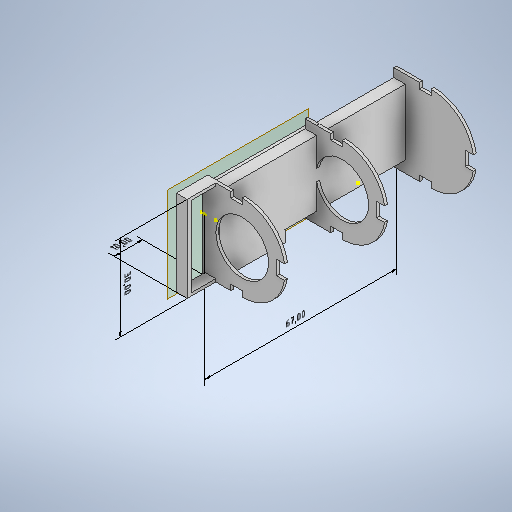
# Autodesk Inventor part: Part4
Saved by Autodesk Inventor 2025.3 (Build 293356000, 356)
## iProperties
Created: 2025-06-07
Part Number: Part4
Material: Generic
Document SubType Name: Modeling
Designer: Repete
Density: 1 g/cm^3
Appearance: Default
Author: Repete
Autodesk Inventor part; units mm, degrees
ref_plane "YZ Plane" through (0, 0, 0) normal (1, 0, 0) x (0, 1, 0)
ref_plane "XZ Plane" through (0, 0, 0) normal (0, 1, 0) x (-1, 0, 0)
ref_plane "XY Plane" through (0, 0, 0) normal (0, 0, 1) x (1, 0, 0)
sketch "Sketch1" plane through (0, 0, 0) normal (0, 1, 0) x (-1, 0, 0)
  circle A0 centre (4.6316, -3.7972) radius 9.2
  line L0 (17.6316, 11.2028) -> (4.6316, 11.2028)
  line L1 (4.6316, -18.7972) -> (17.6316, -18.7972)
  line L2 (17.6316, -18.7972) -> (17.6316, 11.2028)
  arc A1 (4.6316, 11.2028) -> (-10.1586, -1.2972) centre (4.6316, -3.7972) ccw
  arc A2 (-10.1586, -6.2972) -> (4.6316, -18.7972) centre (4.6316, -3.7972) ccw
  arc A3 (-10.1586, -1.2972) -> (-10.1586, -6.2972) centre (4.6316, -3.7972) ccw
  point P0 (17.6316, -3.7972)
  dimension "d6" = 30
  dimension "d7" = 18.4
  dimension "d13" = 13
  constraints: 6 end point, 6 point on circle, 4 centre point, 2 concentric, 1 coincident, 1 horizontal, 1 midpoint, 1 parallel
  measures "d6" distance of L1.end L0.start
  measures "d7" diameter of A0
  measures "d13" distance of point (17.632, -3.797) A0.centre
extrude "Extrusion1" add sketch "Sketch1" along normal blind 1
sketch "Sketch5" plane through (0, 1, 0) normal (0, 1, 0) x (1, 0, 0)
  line L0 (-17.6316, 18.7972) -> (-17.6316, -11.2028) projected
  line L1 (-4.6316, 18.7972) -> (-17.6316, 18.7972) projected
  line L2 (-17.6316, -11.2028) -> (-13.6316, -11.2028)
  line L3 (-13.6316, -11.2028) -> (-13.6316, 18.7972)
  line L4 (-13.6316, 18.7972) -> (-17.6316, 18.7972)
  line L5 (-17.6316, 18.7972) -> (-17.6316, -11.2028)
  point P0 (0, 0)
  dimension "d17" = 4
  constraints: 8 end point, 2 parallel, 1 horizontal, 1 perpendicular, 1 point on line
  measures "d17" distance between parallel lines of L0 L3
extrude "Extrusion2" add sketch "Sketch5" along normal blind 35
sketch "Sketch6" plane through (-17.6316, 0, -18.7972) normal (-1, 0, 0) x (0, 0, 1)
  line L0 (0, 0) -> (0, 36) projected
  line L1 (0, 1) -> (25, 1)
  line L2 (25, 1) -> (25, 35)
  line L3 (25, 35) -> (0, 35)
  line L4 (0, 35) -> (0, 1)
  line L5 (0, 0) -> (30, 0) projected
  point P0 (18.7972, 0)
  point P1 (0, 35)
  point P2 (0, 35)
  dimension "d20" = 25
  dimension "d21" = 1
  dimension "d22" = 34
  constraints: 8 end point, 2 parallel, 1 horizontal, 1 perpendicular, 1 point on line
  measures "d20" distance of L1.start L1.end
  measures "d21" distance between parallel lines of L5 L1
  measures "d22" distance between parallel lines of L1 L3
extrude "Extrusion3" cut sketch "Sketch6" against normal blind 3
sketch "Sketch7" plane through (-17.6316, 0, -18.7972) normal (-1, 0, 0) x (0, 0, 1)
  point P0 (18.7972, 0)
sketch "Sketch8" plane through (-17.6316, 0, -18.7972) normal (-1, 0, 0) x (0, 0, 1)
  line L0 (30, 1) -> (30, 36) projected
  line L1 (25, 35) -> (25, 1) projected
  line L2 (30, 15) -> (25, 15)
  line L3 (25, 15) -> (25, 23)
  line L4 (25, 23) -> (30, 23)
  line L5 (30, 23) -> (30, 15)
  line L6 (0, 0) -> (30, 0) projected
  point P0 (18.7972, 0)
  point P1 (27.5, 15)
  point P2 (27.5, 23)
  point P3 (24, 34.5)
  dimension "d27" = 15
  dimension "d28" = 8
  constraints: 8 end point, 2 midpoint, 2 parallel, 1 horizontal, 1 perpendicular, 1 point on line, 2 other
  measures "d27" distance from line of L6 point (27.5, 15)
  measures "d28" distance of point (27.5, 15) point (27.5, 23)
extrude "Extrusion4" [suppressed]
sketch "Sketch9" plane through (-14.6316, 35, 6.2028) normal (0, 0, -1) x (-1, 0, 0)
  line L0 (3, -12) -> (3.5, -12) projected
  line L1 (3, 0) -> (3, -34) projected
  line L2 (3.5, -12) -> (3, -12)
  line L3 (3, -12) -> (3, -20)
  line L4 (3, -20) -> (3.5, -20)
  line L5 (3.5, -20) -> (3.5, -12)
  point P0 (-14.6316, -35)
  constraints: 8 end point, 2 parallel, 1 horizontal, 1 perpendicular
extrude "Extrusion5" [suppressed]
sketch "Sketch12" plane through (-18.1316, 23, 11.2028) normal (0, 1, 0) x (1, 0, 0)
  line L0 (0, 0) -> (0, 22) projected
  line L1 (0.5, 5) -> (0.5, 22) projected
  line L2 (0, 22) -> (0.5, 22)
  line L3 (0.5, 15.462) -> (0, 15.462)
  line L4 (0, 15.462) -> (0, 22)
  line L5 (0.5, 15.462) -> (1.9334, 18.7689)
  line L6 (1.9334, 18.7689) -> (1.9334, 22)
  line L7 (1.9334, 22) -> (0.5, 22)
  point P0 (18.1316, 11.2028)
  dimension "d36" = 0.5
  constraints: 12 end point, 1 horizontal, 1 parallel, 1 perpendicular, 1 point on line, 1 vertical
  measures "d36" distance of L0.end L2.end
extrude "Extrusion6" [suppressed]
fillet "Fillet1" [suppressed]
sketch "Sketch20" plane through (0, 36, 0) normal (0, 1, 0) x (1, 0, 0)
  point P0 (0, 0)
ref_plane "Work Plane1" through (0, 36, 0) normal (0, -1, 0) x (1, 0, 0)
sketch "Sketch24" plane through (-4.6316, 0, -18.7972) normal (0, 0, -1) x (-1, 0, 0)
  line L0 (0, 0) -> (-14.7902, 0) projected
  line L1 (0, 1) -> (9, 1) projected
  line L2 (0, 0) -> (4, 0)
  line L3 (4, 0) -> (4, 1)
  line L4 (4, 1) -> (0, 1)
  line L5 (0, 1) -> (0, 0)
  point P0 (-4.6316, 0)
  dimension "d69" = 4
  constraints: 8 end point, 2 parallel, 1 horizontal, 1 perpendicular, 1 point on line
  measures "d69" distance between parallel lines of L3 L5
extrude "Extrusion16" cut sketch "Sketch24" against normal blind 2
sketch "Sketch25" plane through (-17.6316, 0, 11.2028) normal (0, 0, 1) x (1, 0, 0)
  line L0 (4, 1) -> (13, 1) projected
  line L1 (3.8, 0) -> (22.2, 0) projected
  line L2 (13, 1) -> (9, 1)
  line L3 (9, 1) -> (9, 0)
  line L4 (9, 0) -> (13, 0)
  line L5 (13, 0) -> (13, 1)
  point P0 (17.6316, 0)
  dimension "d72" = 4
  constraints: 8 end point, 2 parallel, 1 horizontal, 1 perpendicular, 1 point on line
  measures "d72" distance between parallel lines of L3 L5
extrude "Extrusion17" cut sketch "Sketch25" against normal blind 2
sketch "Sketch30" plane through (-13.6316, 1, -1.8894) normal (1, 0, 0) x (0, 0, -1)
  point P0 (-1.8894, -1)
sketch "Sketch31" plane through (-13.6316, 1, -1.8894) normal (1, 0, 0) x (0, 0, -1)
  line L0 (-13.0921, 0) -> (-13.0921, 35) projected
  line L1 (16.9079, 0) -> (-13.0921, 0) projected
  line L2 (-13.0921, 34) -> (-10.0921, 34)
  line L3 (-10.0921, 34) -> (-10.0921, 0)
  line L4 (-10.0921, 0) -> (-13.0921, 0)
  line L5 (-13.0921, 0) -> (-13.0921, 34)
  line L6 (-13.0921, 35) -> (16.9079, 35) projected
  point P0 (-1.8894, -1)
  point P1 (-11.5921, 34)
  dimension "d97" = 3
  dimension "d100" = 1
  constraints: 8 end point, 2 parallel, 2 point on line, 1 horizontal, 1 midpoint, 1 perpendicular
  measures "d97" distance of L2.start L2.end
  measures "d100" distance from line of L6 point (-11.592, 34)
extrude "Extrusion22" cut sketch "Sketch31" against normal through all
sketch "Sketch32" plane through (0, 36, 0) normal (0, -1, 0) x (1, 0, 0)
  circle A0 centre (-4.6552, -3.8036) radius 9.2
  line L0 (-17.6552, -18.8036) -> (-8.6316, -18.8036)
  line L1 (-8.6316, 11.1964) -> (-17.6552, 11.1964)
  line L2 (-17.6552, 11.1964) -> (-17.6552, -18.8036)
  arc A1 (-4.6552, -18.8036) -> (10.135, -6.3036) centre (-4.6552, -3.8036) ccw
  arc A2 (10.135, -6.3036) -> (-4.6552, 11.1964) centre (-4.6552, -3.8036) ccw
  line L3 (-4.6316, 9.2028) -> (-4.6316, 11.2028) projected
  line L4 (-4.6316, 9.2028) -> (-8.6316, 9.2028)
  line L5 (-8.6316, 9.2028) -> (-8.6316, 11.1964)
  line L6 (-4.6316, 11.1964) -> (-4.6316, 9.2028)
  line L7 (-4.6316, -16.7972) -> (-8.6316, -16.7972) projected
  line L8 (-8.6316, -16.7972) -> (-4.6316, -16.7972)
  line L9 (-4.6316, -16.7972) -> (-4.6316, -18.8036)
  line L10 (-8.6316, -18.8036) -> (-8.6316, -16.7972)
  arc A3 (10.135, -6.3036) -> (10.135, -6.3036) centre (-3.0684, -4.0718) ccw
  point P0 (0, 0)
  point P1 (-17.6552, -3.8036)
  point P2 (-4.6316, -16.7972)
  point P3 (10.135, -6.3036)
  dimension "d101" = 30
  dimension "d102" = 18.4
  dimension "d103" = 13
  constraints: 18 end point, 8 point on circle, 4 centre point, 3 parallel, 2 horizontal, 2 perpendicular, 1 coincident, 1 midpoint, 1 tangent
  measures "d101" distance of L1.end L0.start
  measures "d102" diameter of A0
  measures "d103" distance of point (-17.655, -3.804) A0.centre
extrude "Extrusion23" add sketch "Sketch32" along normal blind 1 contours L2 L1 L5 L4 A3 L7 L10 L0 | A3 L4 L3 L9 L7 | A3 A1 L9 | L3 A2 A3
ref_plane "Work Plane3" through (0, 66, 0) normal (0, 1, 0) x (1, 0, 0)
sketch "Sketch34" plane through (0, 66, 0) normal (0, 1, 0) x (1, 0, 0)
  line L0 (-17.6552, -11.1991) -> (-8.6316, -11.1991)
  line L1 (-8.6316, 18.8009) -> (-17.6552, 18.8009)
  line L2 (-17.6552, 18.8009) -> (-17.6552, -11.1991)
  arc A0 (-4.6552, -11.1991) -> (10.135, 1.3009) centre (-4.6552, 3.8009) ccw
  arc A1 (10.135, 6.3009) -> (-4.6552, 18.8009) centre (-4.6552, 3.8009) ccw
  line L3 (-4.6316, 16.8009) -> (-8.6316, 16.8009)
  line L4 (-8.6316, 16.8009) -> (-8.6316, 18.8009)
  line L5 (-4.6316, 18.8009) -> (-4.6316, 16.8009)
  line L6 (-8.6316, -9.1991) -> (-4.6316, -9.1991)
  line L7 (-4.6316, -9.1991) -> (-4.6316, -11.1991)
  line L8 (-8.6316, -11.1991) -> (-8.6316, -9.1991)
  arc A2 (10.135, 1.3009) -> (10.135, 6.3009) centre (-4.6552, 3.8009) ccw
  point P0 (0, 0)
  point P1 (-17.6552, 3.8009)
  dimension "d113" = 30
  dimension "d137" = 2
  dimension "d138" = 2
  constraints: 18 end point, 8 point on circle, 3 centre point, 3 parallel, 2 horizontal, 2 perpendicular, 1 midpoint
  measures "d113" distance of L1.end L0.start
  measures "d137" distance between parallel lines of L6 L0
  measures "d138" distance between parallel lines of L1 L3
extrude "Extrusion25" add sketch "Sketch34" along normal blind 1
sketch "Sketch13" plane through (-14.6316, 0, -18.7972) normal (-1, 0, 0) x (0, 0, 1)
  line L0 (0, 35) -> (25, 35) projected
  line L1 (0, 35) -> (4, 35)
  line L2 (4, 35) -> (4, 24)
  line L3 (4, 24) -> (0, 24)
  line L4 (0, 24) -> (0, 35)
  point P0 (18.7972, 0)
  dimension "d37" = 11
  dimension "d38" = 4
  constraints: 8 end point, 2 parallel, 1 horizontal, 1 perpendicular
  measures "d37" distance of L3.end L0.start
  measures "d38" distance of L2.end L3.end
extrude "Extrusion7" cut sketch "Sketch13" along normal through all both and the other way through all
sketch "Sketch33" plane through (0, 36, 0) normal (0, 1, 0) x (1, 0, 0)
  line L0 (-17.6316, -8.2028) -> (-13.6316, -8.2028)
  line L1 (-13.6316, -8.2028) -> (-13.6316, 14.7972)
  line L2 (-13.6316, 14.7972) -> (-14.6316, 14.7972)
  line L3 (-17.6316, -6.2028) -> (-17.6316, -8.2028)
  line L4 (-17.6316, 18.7972) -> (-17.6316, -11.2028) projected
  line L5 (-17.6316, -6.2028) -> (-14.6316, -6.2028)
  line L6 (-14.6316, -6.2028) -> (-14.6316, 14.7972)
  point P0 (0, 0)
  constraints: 12 end point, 2 horizontal, 2 parallel, 2 perpendicular, 2 other
extrude "Extrusion24" add sketch "Sketch33" along normal up to surface (30 mm away)
sketch "Sketch35" plane through (0, 0, 0) normal (0, -1, 0) x (1, 0, 0)
  line L0 (-17.6316, 11.2028) -> (-8.6316, 11.2028) projected
  line L1 (-17.6316, -18.7972) -> (-14.6316, -18.7972) projected
  line L2 (-13.8651, 11.2028) -> (-17.6316, 11.2028)
  line L3 (-17.6316, 11.2028) -> (-17.6316, -18.7972)
  line L4 (-17.6316, -18.7972) -> (-13.8651, -18.7972)
  line L5 (-13.8651, -18.7972) -> (-13.8651, 11.2028)
  point P0 (0, 0)
  constraints: 8 end point, 2 parallel, 1 horizontal, 1 perpendicular, 1 point on line
extrude "Extrusion26" add sketch "Sketch35" along normal blind 10
sketch "Sketch36" plane through (-13.8651, 0, 11.2028) normal (1, 0, 0) x (0, 0, -1)
  line L0 (0, 0) -> (30, 0) projected
  line L1 (1, 0) -> (29, 0)
  line L2 (29, 0) -> (29, -8.5)
  line L3 (29, -8.5) -> (1, -8.5)
  line L4 (1, -8.5) -> (1, 0)
  line L5 (30, 0) -> (30, -10) projected
  line L6 (0, 0) -> (0, -10) projected
  line L7 (30, -10) -> (0, -10) projected
  point P0 (11.2028, 0)
  point P1 (29, 0)
  dimension "d126" = 1
  dimension "d127" = 1
  dimension "d128" = 1.5
  constraints: 8 end point, 2 parallel, 1 horizontal, 1 perpendicular, 1 point on line
  measures "d126" distance between parallel lines of L5 L2
  measures "d127" distance between parallel lines of L6 L4
  measures "d128" distance between parallel lines of L7 L3
extrude "Extrusion27" cut sketch "Sketch36" against normal through all contours L0 L2 L3 L4
sketch "Sketch37" plane through (0, 67, 0) normal (0, 1, 0) x (1, 0, 0)
  line L0 (12.3499, 1.3009) -> (7.3448, 1.3009)
  line L1 (7.3448, 1.3009) -> (7.3448, 6.3009)
  line L2 (7.3448, 6.3009) -> (12.3499, 6.3009)
  line L3 (12.3499, 6.3009) -> (12.3499, 1.3009)
  arc A0 (-4.6316, -11.1991) -> (-4.6316, 18.8009) centre (-4.6552, 3.8009) ccw projected
  line L4 (-4.6316, 16.8009) -> (-8.6316, 16.8009) projected
  point P0 (0, 0)
  point P1 (12.3499, 3.8009)
  point P2 (9.8474, 1.3009)
  point P3 (9.8474, 6.3009)
  dimension "d140" = 5
  dimension "d143" = 10.5
  dimension "d146" = 12
  constraints: 8 end point, 3 midpoint, 2 parallel, 1 horizontal, 1 perpendicular
  measures "d140" distance between parallel lines of L2 L0
  measures "d143" distance from line of point (9.847, 6.301) L4
  measures "d146" distance from line of A0.centre L1
extrude "Extrusion28" cut sketch "Sketch37" against normal through all
ref_plane "Work Plane4" through (-18.6316, 1, 6.2028) normal (-1, 0, 0) x (0, 0, 1)
sketch "Sketch38" plane through (-18.6316, 1, 6.2028) normal (-1, 0, 0) x (0, 0, 1)
  line L0 (5, -1) -> (-7.5036, -1) projected
  line L1 (-25.0064, 35) -> (1.9936, 35)
  line L2 (1.9936, 35) -> (1.9936, -1)
  line L3 (1.9936, -1) -> (-25.0064, -1)
  line L4 (-25.0064, -1) -> (-25.0064, 35)
  point P0 (-6.2028, -1)
  constraints: 8 end point, 2 parallel, 1 horizontal, 1 perpendicular, 1 point on line
extrude "Extrusion29" add sketch "Sketch38" against normal up to surface (1 mm away)
sketch "Sketch39" plane through (-18.6316, 1, 6.2028) normal (-1, 0, 0) x (0, 0, 1)
  point P0 (-6.2028, -1)
sketch "Sketch40" plane through (-18.6316, 1, 6.2028) normal (-1, 0, 0) x (0, 0, 1)
  line L0 (-25.0064, 34) -> (-21.0064, 34)
  line L1 (-21.0064, 34) -> (-21.0064, 23)
  line L2 (-21.0064, 23) -> (-25.0064, 23)
  line L3 (-25.0064, 23) -> (-25.0064, 34)
  line L4 (-25.0064, 35) -> (-25.0064, -1) projected
  point P0 (-6.2028, -1)
  dimension "d150" = 4
  dimension "d153" = 0
  constraints: 8 end point, 2 parallel, 1 horizontal, 1 perpendicular
  measures "d150" distance of L1.end L2.end
  measures "d153" distance between parallel lines of L4 L3
extrude "Extrusion30" cut sketch "Sketch40" against normal blind 10
sketch "Sketch41" plane through (-18.6316, 1, 6.2028) normal (-1, 0, 0) x (0, 0, 1)
  line L0 (-4.0064, 5) -> (-28.0064, 5)
  line L1 (-28.0064, 5) -> (-28.0064, 30)
  line L2 (-28.0064, 30) -> (-4.0064, 30)
  line L3 (-4.0064, 30) -> (-4.0064, 5)
  line L4 (1.9936, -1) -> (1.9936, 35) projected
  line L5 (1.9936, 35) -> (-25.0064, 35) projected
  line L6 (-25.0064, -1) -> (1.9936, -1) projected
  point P0 (-6.2028, -1)
  dimension "d154" = 24
  dimension "d155" = 6
  dimension "d156" = 5
  dimension "d157" = 6
  constraints: 8 end point, 2 parallel, 1 horizontal, 1 perpendicular
  measures "d154" distance of L1.end L2.end
  measures "d155" distance between parallel lines of L4 L3
  measures "d156" distance between parallel lines of L5 L2
  measures "d157" distance between parallel lines of L6 L0
extrude "Extrusion31" cut sketch "Sketch41" against normal up to surface (1 mm away)
equation "\"d15\" = d45"
equation "\"d45\" = 1"
body "Solid1"
